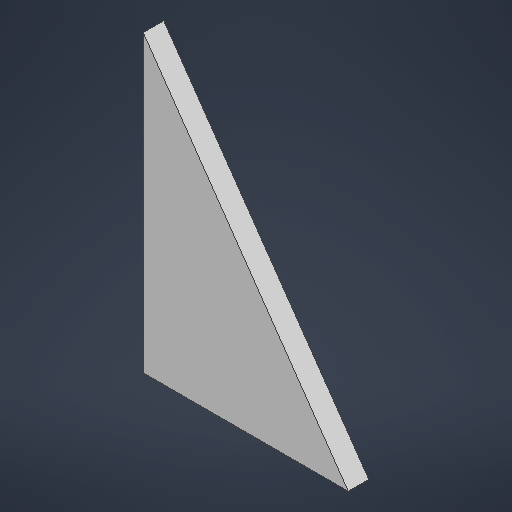
# Autodesk Inventor part: BRACKET GUSSET
Saved by Autodesk Inventor 2025.2 (Build 292293000, 293)
## iProperties
Created: 2025-10-11
Part Number: BRACKET GUSSET
Material: Generic
Document SubType Name: Modeling
Designer: elaij
Density: 1 g/cm^3
Appearance: Default
Author: elaij
Autodesk Inventor part; units mm, degrees
ref_plane "YZ Plane" through (0, 0, 0) normal (1, 0, 0) x (0, 1, 0)
ref_plane "XZ Plane" through (0, 0, 0) normal (0, 1, 0) x (-1, 0, 0)
ref_plane "XY Plane" through (0, 0, 0) normal (0, 0, 1) x (1, 0, 0)
sketch "Sketch1" plane through (0, 0, 0) normal (0, 0, 1) x (1, 0, 0)
  line L0 (0, 0) -> (0, 115)
  line L1 (0, 115) -> (80, 0)
  line L2 (80, 0) -> (0, 0)
  dimension "d0" = 115
  dimension "d1" = 80
  constraints: 6 end point, 1 perpendicular, 1 vertical
  measures "d0" distance of L0.start L0.end
  measures "d1" distance of L1.end L0.start
extrude "Extrusion1" add sketch "Sketch1" against normal blind 8
body "Solid1"
